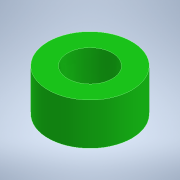
# Autodesk Inventor part: motor-mount-bottom
Saved by Autodesk Inventor 2021 (Build 250183000, 183)
## iProperties
Created: 2021-03-30
Part Number: motor-mount-bottom
Material: ABS Plastic
Document SubType Name: Modeling
Designer: samlo
Density: 1.06 g/cm^3
Appearance: Dark Green
Author: samlo
Autodesk Inventor part; units mm, degrees
ref_plane "YZ Plane" through (0, 0, 0) normal (1, 0, 0) x (0, 1, 0)
ref_plane "XZ Plane" through (0, 0, 0) normal (0, 1, 0) x (-1, 0, 0)
ref_plane "XY Plane" through (0, 0, 0) normal (0, 0, 1) x (1, 0, 0)
sketch "Sketch1" plane through (0, 0, 0) normal (0, 0, 1) x (1, 0, 0)
  line L0 (13.335, 0) -> (25, 0)
  line L1 (25, 0) -> (25, 25)
  line L2 (25, 25) -> (13.335, 25)
  line L3 (13.335, 25) -> (13.335, 0)
  line L4 (0, -5) -> (0, 30) projected
  point P0 (0, 0)
  dimension "d0" = 13.335
  dimension "d1" = 25
  dimension "d2" = 25
  dimension "d3" = 11.665
  constraints: 8 end point, 3 perpendicular, 1 horizontal
  measures "d0" distance of L0.start point (0, 0)
  measures "d1" distance of L0.end point (0, 0)
  measures "d2" vertical distance of L2.end point (0, 0)
  measures "d3" distance between parallel lines of L1 L3
revolve "Revolution1" add sketch "Sketch1" angle 360 about axis through (0, -10, 0) along (0, 1, 0)
body "Solid1"
